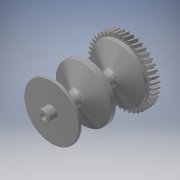
# Autodesk Inventor part: Spur Gear2
Saved by Autodesk Inventor 2019 (Build 230136000, 136)
## iProperties
Created: 2020-07-29
Part Number: Spur Gear2
Material: Steel
Document SubType Name: Modeling
Designer: Ian
Categories: <?xml version="1.0" encoding="UTF-16"?> <MemberInstance><Categories><FamilyTemplate><FamilyTemplateParameter ValueType="xs:double" Id="1" ObjectReferenceKey="da_z" ObjectType="kUserParameterObject"/><FamilyTemplateParameter ValueType="xs:double" Id="2" ObjectReferenceKey="da_b" ObjectType="kUserParameterObject"/><FamilyTemplateParameter ValueType="xs:double" Id="3" ObjectReferenceKey="da_beta" ObjectType="kUserParameterObject"/><FamilyTemplateParameter ValueType="xs:double" Id="4" ObjectReferenceKey="da_da" ObjectType="kUserParameterObject"/><FamilyTemplateParameter ValueType="xs:double" Id="5" ObjectReferenceKey="da_aw" ObjectType="kUserParameterObject"/><FamilyTemplateParameter ValueType="xs:string" Id="6" ObjectReferenceKey="EAIAABAAAACIAQAAAAAAAIAAAAAAAAAA" ObjectType="83910656" SubObjectId="SurfaceGeometry"/></FamilyTemplate><ParamToTemplateMap><ParamToTemplate CategoryParameter="//CategoryParameter[@InternalName='046C89C9-8512-4d59-83FE-43B91F4F132A']" TemplateParameter="1"/><ParamToTemplate CategoryParameter="//CategoryParameter[@InternalName='2552DF32-E462-4b46-AEBF-C6C7768E72AC']" TemplateParameter="2"/><ParamToTemplate CategoryParameter="//CategoryParameter[@InternalName='C9EE641D-15FC-4fae-A226-E94C4372FDD7']" TemplateParameter="3"/><ParamToTemplate><ParamToTemplate CategoryParameter="//CategoryParameter[@InternalName='00B6519A-459B-49c7-AD84-2E56D39A5744']" ConstantValue="0.281867"/></ParamToTemplate><ParamToTemplate><ParamToTemplate CategoryParameter="//CategoryParameter[@InternalName='04B31F0E-C7A6-4894-AA32-9629BEFACF47']" ConstantValue="1.000000"/></ParamToTemplate><ParamToTemplate><ParamToTemplate CategoryParameter="//CategoryParameter[@InternalName='43CBEC2E-7847-49e7-A936-2F7889FCB2D9']" ConstantValue="0.250000"/></ParamToTemplate><ParamToTemplate><ParamToTemplate CategoryParameter="//CategoryParameter[@InternalName='B1EFC894-105D-4ebd-86BF-FA20ED196853']" ConstantValue="0.350000"/></ParamToTemplate><ParamToTemplate><ParamToTemplate CategoryParameter="//CategoryParameter[@InternalName='51175063-3D10-4879-93E8-6246FE8B403D']" ConstantValue="2060000000.000000"/></ParamToTemplate><ParamToTemplate><ParamToTemplate CategoryParameter="//CategoryParameter[@InternalName='A3A52E27-4454-46a9-B0BD-C932399B70AF']" ConstantValue="0.300000"/></ParamToTemplate><ParamToTemplate><ParamToTemplate CategoryParameter="//CategoryParameter[@InternalName='91B76062-C214-41d9-B1B9-14D2AB99603D']" ConstantValue="0.050000"/></ParamToTemplate><ParamToTemplate><ParamToTemplate CategoryParameter="//CategoryParameter[@InternalName='374E806E-8B8A-4dda-A9AA-1039D6500AD2']" ConstantValue="20.000000"/></ParamToTemplate><ParamToTemplate><ParamToTemplate CategoryParameter="//CategoryParameter[@InternalName='2D373A89-B862-43d6-8D0B-0CBF12AB9F6C']" ConstantValue="0.349066"/></ParamToTemplate><ParamToTemplate CategoryParameter="//CategoryParameter[@InternalName='37777632-D6A2-4fac-9D53-DB8ACD95C989']" TemplateParameter="4"/><ParamToTemplate CategoryParameter="//CategoryParameter[@InternalName='FD1017F1-B727-4f7e-9707-0F86F1FF9423']" TemplateParameter="5"/><ParamToTemplate><ParamToTemplate CategoryParameter="//CategoryParameter[@InternalName='9E1B4470-B2D3-4ff1-B813-535BB4CDF51A']" ConstantValue="3520000.000000"/></ParamToTemplate><ParamToTemplate><ParamToTemplate CategoryParameter="//CategoryParameter[@InternalName='F8452263-BFF6-458c-9FB1-07C4B99E95CD']" ConstantValue="11400000.000000"/></ParamToTemplate><ParamToTemplate><ParamToTemplate CategoryParameter="//CategoryParameter[@InternalName='3E3BB259-FD49-497f-8171-6EBC954A3479']" ConstantValue="2.000000"/></ParamToTemplate><ParamToTemplate CategoryParameter="//CategoryParameter[@InternalName='27C3BAF2-7550-4e4b-AE2C-0DB134B7D9B7']" TemplateParameter="6"/></ParamToTemplateMap><Category DisplayName="Gear" InternalName="DC85795E-93AB-48d5-8EEE-5A27447B64BD" Mnemonic="Gear"><CategoryParameter DisplayName="z" InternalName="046C89C9-8512-4d59-83FE-43B91F4F132A" Mnemonic="z"/><CategoryParameter DisplayName="b" InternalName="2552DF32-E462-4b46-AEBF-C6C7768E72AC" Mnemonic="b"/><CategoryParameter DisplayName="||b|" InternalName="C9EE641D-15FC-4fae-A226-E94C4372FDD7" Mnemonic="beta"/><CategoryParameter DisplayName="x" InternalName="00B6519A-459B-49c7-AD84-2E56D39A5744" Mnemonic="x"/><CategoryParameter DisplayName="a*" InternalName="04B31F0E-C7A6-4894-AA32-9629BEFACF47" Mnemonic="a"/><CategoryParameter DisplayName="c*" InternalName="43CBEC2E-7847-49e7-A936-2F7889FCB2D9" Mnemonic="c"/><CategoryParameter DisplayName="r|.f|*" InternalName="B1EFC894-105D-4ebd-86BF-FA20ED196853" Mnemonic="rf"/><CategoryParameter DisplayName="E" InternalName="51175063-3D10-4879-93E8-6246FE8B403D" Mnemonic="E"/><CategoryParameter DisplayName="||m|" InternalName="A3A52E27-4454-46a9-B0BD-C932399B70AF" Mnemonic="mi"/><Category DisplayName="SpurGear" InternalName="26C5A22E-A91E-4dfd-A3B3-23CCAFAE1764" Mnemonic="SpurGear"><CategoryParameter DisplayName="m" InternalName="91B76062-C214-41d9-B1B9-14D2AB99603D" Mnemonic="m"/><CategoryParameter DisplayName="P" InternalName="374E806E-8B8A-4dda-A9AA-1039D6500AD2" Mnemonic="PP"/><CategoryParameter DisplayName="||a|" InternalName="2D373A89-B862-43d6-8D0B-0CBF12AB9F6C" Mnemonic="alpha"/><CategoryParameter DisplayName="d|.a|" InternalName="37777632-D6A2-4fac-9D53-DB8ACD95C989" Mnemonic="da"/><CategoryParameter DisplayName="a|.w|" InternalName="FD1017F1-B727-4f7e-9707-0F86F1FF9423" Mnemonic="aw"/><CategoryParameter DisplayName="||s||.Flim|" InternalName="9E1B4470-B2D3-4ff1-B813-535BB4CDF51A" Mnemonic="sFlim"/><CategoryParameter DisplayName="||s||.Hlim|" InternalName="F8452263-BFF6-458c-9FB1-07C4B99E95CD" Mnemonic="sHlim"/><CategoryParameter DisplayName="type" InternalName="3E3BB259-FD49-497f-8171-6EBC954A3479" Mnemonic="type"/><CategoryParameter DisplayName="PitchDiameter" InternalName="27C3BAF2-7550-4e4b-AE2C-0DB134B7D9B7" Mnemonic="IDS_PITCHDIAM"/></Category></Category></Categories></MemberInstance>
Density: 1 g/cm^3
Appearance: Steel
CustomPartVersion: 1
Author: Ian
Autodesk Inventor part; units mm, degrees
sketch "Sketch1" plane through (0, 0, 0) normal (0, 0, 1) x (1, 0, 0)
  circle A0 centre (0, 0) radius 11.6271
  dimension "d0" = 23.2542
  constraints: 1 centre point
  measures "d0" diameter of A0
extrude "Extrusion1" add sketch "Sketch1" along normal blind 3
ref_plane "Work Plane2" through (0, 0, 1.5) normal (0, 0, 1) x (1, 0, 0)
sketch "Sketch2" plane through (0, 0, 0) normal (0, 0, -1) x (-1, 0, 0)
  circle A0 centre (0, 0) radius 11.6271 projected
  circle A1 centre (0, 0) radius 11.0808
  dimension "d3" = 22.1615
  constraints: 1 centre point, 1 coincident
  measures "d3" diameter of A1
surface extrude "Pitch Diameter" sketch "Sketch2" against normal through all shown no curves A1
ref_plane "Work Plane8" through (0, 0, 0) normal (0.9973323, 0.0729953, 0) x (0, 0, 1)
ref_plane "Work Plane9" through (0, 0, 0) normal (1, 0, 0) x (0, 1, 0)
spur gear teeth "Spur Gear" teeth 43 pitch diameter 21.9803 tip diameter 23.2543 root diameter 21.0122 face width 3 helix angle 12 hand right start plane through (0, 0, 0) normal (0, 0, -1) x (-1, 0, 0)
sketch "Sketch3" plane through (0, 0, 0) normal (1, 0, 0) x (0, 1, 0)
  line L0 (-10, 3) -> (-10, 28) projected
  line L1 (10, 28) -> (10, 3) projected
  line L2 (-10, 28) -> (10, 28) projected
  line L3 (10, 3) -> (-10, 3) projected
  line L4 (-10, 3) -> (-10, 4)
  line L5 (-10, 4) -> (-2.25, 6.8208)
  line L6 (0, -35.2538) -> (0, 68.4313) projected
  line L7 (-2.25, 3) -> (-2.25, 28)
  line L8 (-10, 28) -> (-10, 27)
  line L9 (-10, 27) -> (-2.25, 24.1792)
  line L10 (-10, 15.5) -> (-5.6858, 15.5)
  line L11 (-10, 15.5) -> (-10, 14.5)
  line L12 (-10, 14.5) -> (-2.25, 11.6792)
  line L13 (-10, 15.5) -> (-10, 16.5)
  line L14 (-10, 16.5) -> (-2.25, 19.3208)
  point P0 (0, 0)
  dimension "d49" = 1
  dimension "d50" = 110
  dimension "d53" = 2.25
  dimension "d55" = 1
  dimension "d56" = 110
  dimension "d57" = 1
  dimension "d58" = 110
  dimension "d59" = 1
  dimension "d60" = 110
  constraints: 20 end point, 10 point on line, 2 midpoint, 1 horizontal, 1 parallel
  measures "d49" distance of L0.start L4.end
  measures "d50" angle of L4 L5
  measures "d53" distance between parallel lines of L6 L7
  measures "d55" distance of L0.end L8.end
  measures "d56" angle of L9 L8
  measures "d57" distance of L10.start L11.end
  measures "d58" angle of L12 L11
  measures "d59" distance of L10.start L13.end
  measures "d60" angle of L13 L14
revolve "Revolution1" add sketch "Sketch3" angle 360 about axis through (0, 0, -35.2538) along (0, 0, 1) contours L0 L5 L7 L3 | L0 L14 L7 L12 | L7 L9 L0 L2
sketch "Sketch4" plane through (0, 0, 3) normal (0, 0, 1) x (1, 0, 0)
  circle A0 centre (0, 0) radius 2.25 projected
  circle A1 centre (0, 0) radius 3
  point P0 (0, 0)
  dimension "d72" = 4.5
  dimension "d73" = 0.75
  constraints: 1 centre point
  measures "d72" diameter of A0
  measures "d73" radial gap between concentric circles of A0 A1
extrude "Extrusion2" add sketch "Sketch4" along normal up to surface (25 mm away) contours A0 | A1
fillet "Fillet1" radius 1.5 8 edges at (-2.1213, 2.1213, 6.5478) (2.1213, -2.1213, 6.5478) (-2.1213, 2.1213, 19.0478) (2.1213, -2.1213, 19.0478) (2.1213, -2.1213, 24.4522) (-2.1213, 2.1213, 24.4522) (2.1213, -2.1213, 11.9522) (-2.1213, 2.1213, 11.9522)
sketch "Sketch5" plane through (0, 0, 0) normal (0, 0, -1) x (-1, 0, 0)
  circle A0 centre (0, 0) radius 2.5
  dimension "d65" = 5
  constraints: 1 centre point, 1 coincident
  measures "d65" diameter of A0
extrude "Extrusion3" add sketch "Sketch5" along normal blind 3
fillet "Fillet2" radius 0.25 6 edges at (0, 10, 4) (0, 10, 14.5) (0, 10, 16.5) (0, 10, 28) (0, 10, 27) (2.5, 0, -3)
sketch "Sketch6" plane through (0, 0, -3) normal (0, 0, -1) x (-1, 0, 0)
  circle A0 centre (0, 0) radius 1.05
  dimension "d69" = 2.1
  constraints: 1 centre point, 1 coincident
  measures "d69" diameter of A0
extrude "Extrusion4" cut sketch "Sketch6" along normal through all both and the other way through all
sketch "Sketch7" plane through (0, 0, 28) normal (0, 0, 1) x (1, 0, 0)
  circle A0 centre (0, 0) radius 1.05 projected
  circle A1 centre (0, 0) radius 2.25
  point P0 (0, 0)
  dimension "d74" = 4.5
  constraints: 1 centre point, 1 coincident
  measures "d74" diameter of A1
ref_plane "Work Plane11" through (-11.25, -4, 31.15) normal (0, 0, 1) x (1, 0, 0)
extrude "Extrusion5" add sketch "Sketch7" along normal up to surface (3.15 mm away)
fillet "Fillet3" radius 0.25 1 edges at (-2.25, 0, 31.15)
sketch "Sketch8" plane through (0, 0, 0) normal (0, 0, -1) x (-1, 0, 0)
  line L0 (0, -5.7735) -> (-5, 2.8868)
  line L1 (-5, 2.8868) -> (5, 2.8868)
  line L2 (5, 2.8868) -> (0, -5.7735)
  circle A0 centre (0, -5.7735) radius 1.05
  circle A1 centre (-5, 2.8868) radius 1.05
  circle A2 centre (5, 2.8868) radius 1.05
  point P0 (0, 0)
  point P1 (0, 0)
  dimension "d78" = 10
  dimension "d79" = 2.1
  dimension "d80" = 2.1
  dimension "d81" = 2.1
  constraints: 6 end point, 4 coincident, 3 centre point, 1 horizontal, 7 other
  measures "d78" distance of L0.end L1.end
  measures "d79" diameter of A0
  measures "d80" diameter of A1
  measures "d81" diameter of A2
extrude "Extrusion6" cut sketch "Sketch8" against normal up to surface contours L2 A0 L0 | L0 A0 L2 | A1 L1 L0 | L0 L1 A1 | A2 L1 L2 | L2 L1 A2 round surface about axis through (0, 0, 13.0896) along (0, 0, 1) radius 6.125 half angle 70 far side no
equation "\"d0\" = da_da"
equation "\"d1\" = da_b"
equation "\"d3\" = da_dw"
equation "\"d16\" = da_aw"
equation "\"d43\" = da_aw"
equation "\"d46\" = da_aw"
equation "\"da_da\" = 23.254253"
equation "\"da_b\" = 3"
equation "\"da_dw\" = 22.161538"
equation "\"da_aw\" = 16.75"
body "Solid1"
body "Srf1"
